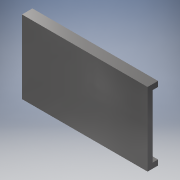
# Autodesk Inventor part: Soporte_rods
Saved by Autodesk Inventor 2018 (Build 220112000, 112)
## iProperties
Created: 2021-07-05
Part Number: Soporte_rods
Material: Acero, fundido
Document SubType Name: Modeling
Designer: GABRIEL
Density: 7.85 g/cm^3
Appearance: Semipulido
Author: GABRIEL
Autodesk Inventor part; units mm, degrees
ref_plane "YZ Plane" through (0, 0, 0) normal (1, 0, 0) x (0, 1, 0)
ref_plane "XZ Plane" through (0, 0, 0) normal (0, 1, 0) x (-1, 0, 0)
ref_plane "XY Plane" through (0, 0, 0) normal (0, 0, 1) x (1, 0, 0)
sketch "Boceto1" plane through (0, 0, 0) normal (0, 1, 0) x (-1, 0, 0)
  line L0 (0, 0) -> (-200, 0)
  line L1 (-200, 0) -> (-200, -140)
  line L2 (-200, -140) -> (0, -140)
  line L3 (0, -140) -> (0, 0)
  line L4 (0, 0) -> (-200, 0)
  line L5 (-200, 0) -> (-200, -10)
  line L6 (-200, -10) -> (0, -10)
  line L7 (0, -10) -> (0, 0)
  line L8 (0, -140) -> (-200, -140)
  line L9 (-200, -140) -> (-200, -130)
  line L10 (-200, -130) -> (0, -130)
  line L11 (0, -130) -> (0, -140)
  dimension "d0" = 200
  dimension "d1" = 140
  dimension "d2" = 200
  dimension "d3" = 10
  dimension "d4" = 200
  dimension "d5" = 10
  constraints: 24 end point, 6 parallel, 3 horizontal, 3 perpendicular
  measures "d0" distance of L2.end L1.end
  measures "d1" distance of L1.end L0.end
  measures "d2" distance of L6.end L5.end
  measures "d3" distance of L5.end L4.end
  measures "d4" distance of L9.end L10.end
  measures "d5" distance of L8.end L9.end
extrude "Extrusión1" add sketch "Boceto1" along normal blind 10 contours L3 L10 L1 L6
extrude "Extrusión2" add sketch "Boceto1" along normal blind 70 contours L3 L6 L1 L0 | L3 L2 L1 L10
